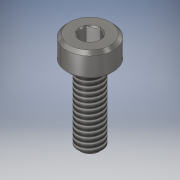
# Autodesk Inventor part: Bolt_M2x0.4_6mm_SH
Saved by Autodesk Inventor 2018 (Build 220112000, 112)
## iProperties
Manager: Bradley
Company: Zetta & Zepto Technology
Created: 2016-07-03
Part Number: Bolt_M2x0.4_6mm_SH
Material: Stainless Steel
Document SubType Name: Modeling
Designer: Bradley
Density: 8 g/cm^3
Appearance: Semi-Polished
Description: SCM4006-3H3
Stock Number: 80110
Author: Bradley
Autodesk Inventor part; units mm, degrees
ref_plane "YZ Plane" through (0, 0, 0) normal (1, 0, 0) x (0, 1, 0)
ref_plane "XZ Plane" through (0, 0, 0) normal (0, 1, 0) x (-1, 0, 0)
ref_plane "XY Plane" through (0, 0, 0) normal (0, 0, 1) x (1, 0, 0)
sketch "Sketch1" plane through (0, 0, 0) normal (0, 0, 1) x (1, 0, 0)
  line L0 (0, 4) -> (0, -4)
  line L1 (0, -4) -> (0.75, -4)
  line L2 (0.75, -4) -> (1, -3.75)
  line L3 (1, -3.75) -> (1, 1.9)
  line L4 (1.1, 2) -> (1.65, 2)
  line L5 (1.9, 2.25) -> (1.9, 3.75)
  line L6 (1.65, 4) -> (0, 4)
  arc A0 (1.1, 2) -> (1, 1.9) centre (1.1, 1.9) ccw
  line L7 (1.65, 4) -> (1.9, 3.75)
  line L8 (1.65, 2) -> (1.9, 2.25)
  point P0 (0, 0)
  point P1 (1.9, 2)
  point P2 (1.9, 4)
  point P3 (0, 0)
  dimension "d0" = 3.8
  dimension "d1" = 2
  dimension "d3" = 2
  dimension "d4" = 2.2
  dimension "d5" = 135
  dimension "d6" = 0.25
  dimension "d7" = 6
  dimension "d18" = 0.25
  constraints: 18 end point, 6 perpendicular, 6 point on line, 2 point on circle, 2 tangent, 1 centre point, 1 coincident, 1 midpoint, 1 parallel, 1 vertical, 1 vertical alignment
  measures "d0" diameter of L5 L0
  measures "d1" distance of point (1.9, 2) point (1.9, 4)
  measures "d3" diameter of L3 L0
  measures "d4" diameter of L4.start L0
  measures "d5" angle of L3 L2
  measures "d6" horizontal distance of L1.end L2.end
  measures "d7" distance between parallel lines of L1 L4
  measures "d18" distance of L6.start point (1.9, 4)
revolve "Revolution1" add sketch "Sketch1" angle 360 about axis through (0, 4, 0) along (0, -1, 0)
sketch "Sketch2" plane through (0, 4, 0) normal (0, 1, 0) x (1, 0, 0)
  line L0 (0, -0.866) -> (-0.75, -0.433)
  line L1 (-0.75, -0.433) -> (-0.75, 0.433)
  line L2 (-0.75, 0.433) -> (0, 0.866)
  line L3 (0, 0.866) -> (0.75, 0.433)
  line L4 (0.75, 0.433) -> (0.75, -0.433)
  line L5 (0.75, -0.433) -> (0, -0.866)
  point P0 (0, 0)
  point P1 (0, 0)
  dimension "d11" = 1.5
  constraints: 12 end point, 1 coincident, 1 vertical, 13 other
  measures "d11" distance between parallel lines of L4 L1
extrude "Extrusion1" cut sketch "Sketch2" against normal blind 1.5
thread "Thread1" size "M2x0.4" class "6g" standard "ANSI Metric M Profile" full length
sketch "Sketch3" plane through (0, 0, 0) normal (1, 0, 0) x (0, 1, 0)
  line L0 (4, 0.866) -> (4, 0.433) projected
  line L1 (4, 0.866) -> (3.5, 0.366)
  line L2 (3.5, 0.366) -> (4, 0.366)
  line L3 (4, 0.366) -> (4, 0.866)
  line L4 (-0.8, 0) -> (4.8, 0) projected
  point P0 (0, 0)
  dimension "d16" = 0.5
  constraints: 6 end point, 3 perpendicular
  measures "d16" distance of L2.end L0.start
revolve "Revolution2" cut sketch "Sketch3" angle 360 about axis through (0, -10, 0) along (0, 1, 0)
body "Solid1"
